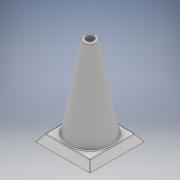
# Autodesk Inventor part: mini_corn
Saved by Autodesk Inventor 2018.2 (Build 222227000, 227)
## iProperties
Created: 2017-12-15
Part Number: mini_corn
Material: 一般
Document SubType Name: Modeling
Designer: ku_sk
Density: 1 g/cm^3
Appearance: 既定
Author: ku_sk
## iProperties of the stored document mini_corn_3D プリント.ipt
Created: 2017-12-15
Part Number: mini_corn_3D プリント
Material: 一般
Document SubType Name: Modeling
Designer: ku_sk
Density: 1 g/cm^3
Appearance: 既定
Author: ku_sk
Autodesk Inventor part; units mm, degrees
ref_plane "YZ Plane" through (0, 0, 0) normal (1, 0, 0) x (0, 1, 0)
ref_plane "XZ Plane" through (0, 0, 0) normal (0, 1, 0) x (-1, 0, 0)
ref_plane "XY Plane" through (0, 0, 0) normal (0, 0, 1) x (1, 0, 0)
sketch "スケッチ1" plane through (0, 0, 0) normal (1, 0, 0) x (0, 1, 0)
  line L0 (0, 0) -> (105, 0)
  line L1 (105, 0) -> (31.5, 415)
  line L2 (31.5, 415) -> (0, 415)
  line L3 (0, 415) -> (0, 0)
  dimension "d0" = 415
  dimension "d1" = 31.5
  dimension "d2" = 105
  constraints: 8 end point, 1 horizontal, 1 parallel, 1 perpendicular
  measures "d0" distance of L2.end L0.start
  measures "d1" distance of L1.end L2.end
  measures "d2" distance of L0.start L0.end
revolve "回転1" add sketch "スケッチ1" angle 360 about axis through (0, 0, 415) along (0, 0, -1)
sketch "スケッチ2" plane through (0, 0, 0) normal (0, 0, -1) x (-1, 0, 0)
  line L0 (-137.5, -137.5) -> (137.5, -137.5)
  line L1 (137.5, -137.5) -> (137.5, 137.5)
  line L2 (137.5, 137.5) -> (-137.5, 137.5)
  line L3 (-137.5, 137.5) -> (-137.5, -137.5)
  line L4 (-137.5, -137.5) -> (137.5, 137.5) construction
  line L5 (137.5, -137.5) -> (-137.5, 137.5) construction
  point P0 (0, 0)
  dimension "d4" = 275
  dimension "d5" = 275
  constraints: 12 end point, 2 midpoint, 2 parallel, 1 horizontal, 1 perpendicular
  measures "d4" distance of L2.end L0.start
  measures "d5" distance of L1.end L2.end
extrude "押し出し1" add sketch "スケッチ2" along normal blind 35
chamfer "面取り3" distance 35 distance2 25 1 edges at (0, 137.5, 0) measured on face at (-45.8333, 137.5, -11.6667)
chamfer "面取り4" distance 35 distance2 25 1 edges at (137.5, -12.5, 0) measured on face at (137.5, 37.5, -23.3333)
chamfer "面取り5" distance 35 distance2 25 1 edges at (-12.5, -137.5, 0) measured on face at (37.5, -137.5, -23.3333)
chamfer "面取り6" distance 35 distance2 25 1 edges at (-137.5, 0, 0) measured on face at (-137.5, -37.5, -23.3333)
shell "シェル1" thickness 11.5 removed faces 2 at (9.3296, 8.757, 415) at (45.8333, -45.8333, -35)
fillet "フィレット2" radius 5 19 edges at (0, -31.5, 415) (112.5001, 0, 0) (0, -112.5001, 0) (125, -125.0001, -17.5) (0, -105, 0) (125.0001, 125, -17.5) (0, 112.5001, 0) (-112.5001, 0, 0) (-125.0001, 125, -17.4999) (-125.0001, -125, -17.5) (0, -95.3578, -11.5) (0, -106.582, -11.5) (-106.582, 0, -11.5) (-114.9748, -114.9748, -23.25) (0, 106.582, -11.5) (106.582, 0, -11.5) (114.9748, 114.9748, -23.25) (-114.9748, 114.9748, -23.25) (114.9748, -114.9748, -23.25)
equation "\"d5\" = d4"
